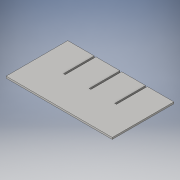
# Autodesk Inventor part: Wine Rack Horizontal
Saved by Autodesk Inventor 2016 (Build 200138000, 138)
## iProperties
Created: 2017-10-31
Part Number: Wine Rack Horizontal
Material: Generic
Document SubType Name: Modeling
Designer: mathaetaes
Density: 1 g/cm^3
Appearance: Default
Author: mathaetaes
Autodesk Inventor part; units mm, degrees
ref_plane "YZ Plane" through (0, 0, 0) normal (1, 0, 0) x (0, 1, 0)
ref_plane "XZ Plane" through (0, 0, 0) normal (0, 1, 0) x (-1, 0, 0)
ref_plane "XY Plane" through (0, 0, 0) normal (0, 0, 1) x (1, 0, 0)
sketch "Sketch1" plane through (0, 0, 0) normal (0, 1, 0) x (-1, 0, 0)
  line L0 (163.957, -96.9264) -> (-229.743, -96.9264)
  line L1 (-229.743, -96.9264) -> (-229.743, 131.6736)
  line L2 (-229.743, 131.6736) -> (163.957, 131.6736)
  line L3 (163.957, 131.6736) -> (163.957, -96.9264)
  point P0 (0, 0)
  dimension "d0" = 228.6
  dimension "d1" = 393.7
  constraints: 8 end point, 2 parallel, 1 horizontal, 1 perpendicular
  measures "d0" distance of L0.end L1.end
  measures "d1" distance of L0.start L0.end
extrude "Board" add sketch "Sketch1" along normal blind 6.35
sketch "Sketch2" plane through (0, 6.35, 0) normal (0, 1, 0) x (1, 0, 0)
  line L0 (-65.532, 96.9264) -> (-59.182, 96.9264)
  line L1 (-59.182, 96.9264) -> (-59.182, -17.3736)
  line L2 (-59.182, -17.3736) -> (-65.532, -17.3736)
  line L3 (-65.532, -17.3736) -> (-65.532, 96.9264)
  line L4 (229.743, 96.9264) -> (-163.957, 96.9264) projected
  line L5 (-163.957, 96.9264) -> (-163.957, -131.6736) projected
  line L6 (29.718, 96.9264) -> (36.068, 96.9264)
  line L7 (36.068, 96.9264) -> (36.068, -17.3736)
  line L8 (36.068, -17.3736) -> (29.718, -17.3736)
  line L9 (29.718, -17.3736) -> (29.718, 96.9264)
  line L10 (124.968, 96.9264) -> (131.318, 96.9264)
  line L11 (131.318, 96.9264) -> (131.318, -17.3736)
  line L12 (131.318, -17.3736) -> (124.968, -17.3736)
  line L13 (124.968, -17.3736) -> (124.968, 96.9264)
  line L14 (229.743, -131.6736) -> (229.743, 96.9264) projected
  point P0 (0, 0)
  dimension "d4" = 6.35
  dimension "d5" = 114.3
  dimension "d6" = 98.425
  dimension "d7" = 6.35
  dimension "d8" = 114.3
  dimension "d10" = 6.35
  dimension "d11" = 114.3
  dimension "d13" = 88.9
  dimension "d14" = 88.9
  dimension "d25" = 98.425
  constraints: 24 end point, 6 parallel, 3 horizontal, 3 perpendicular, 1 collinear
  measures "d4" distance of L0.start L0.end
  measures "d5" distance of L2.end L0.start
  measures "d6" distance between parallel lines of L5 L3
  measures "d7" distance of L6.start L6.end
  measures "d8" distance of L8.end L6.start
  measures "d10" distance of L10.start L10.end
  measures "d11" distance of L12.end L10.start
  measures "d13" distance between parallel lines of L9 L1
  measures "d14" distance between parallel lines of L13 L7
  measures "d25" distance between parallel lines of L14 L11
extrude "Stop Dados" cut sketch "Sketch2" against normal blind 6.35
equation "\"d5\" = 0.5 * d0"
equation "\"d8\" = 0.5 * d9"
equation "\"d11\" = 0.5 * d12"
equation "\"d9\" = 228.6"
equation "\"d12\" = 228.6"
body "Solid1"
